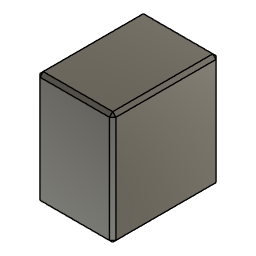
Battery Box v3 (Autodesk Fusion 360 design; units mm, degrees)
Autodesk Fusion 360 part; units mm, degrees
sketch "Sketch1" plane through (0, 0, 0) normal (0, 0, 1) x (1, 0, 0)
  line L0 (0, 0) -> (47, 0)
  line L1 (47, 0) -> (47, 66)
  line L2 (47, 66) -> (0, 66)
  line L3 (0, 66) -> (0, 0)
  dimension "d1" = 47
  dimension "d2" = 66
  constraint horizontal L0
  constraint vertical L1
  constraint horizontal L2
  constraint vertical L3
  constraint coincident L0.start L3.end
  measures "d1" distance of L0.start L0.end
  measures "d2" distance of L0.start L2.end
extrude "Extrude1" add sketch "Sketch1" along normal blind 70
chamfer "Chamfer1" distance 2 angle 45 6 faces at (15.6667, 44, 70) (15.6667, 0, 23.3333) (47, 22, 23.3333) (0, 44, 23.3333) (31.3333, 66, 23.3333) (15.6667, 44, 0)
